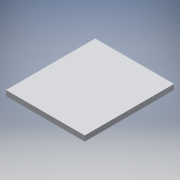
# Autodesk Inventor part: RSX Top
Saved by Autodesk Inventor 2016 (Build 200138000, 138)
## iProperties
Created: 2016-10-30
Part Number: RSX Top
Material: Aluminum 6061
Document SubType Name: Modeling
Designer: eschr_000
Density: 2.7 g/cm^3
Appearance: Aluminum - Flat
Author: eschr_000
Autodesk Inventor part; units mm, degrees
ref_plane "YZ Plane" through (0, 0, 0) normal (1, 0, 0) x (0, 1, 0)
ref_plane "XZ Plane" through (0, 0, 0) normal (0, 1, 0) x (-1, 0, 0)
ref_plane "XY Plane" through (0, 0, 0) normal (0, 0, 1) x (1, 0, 0)
sketch "Sketch1" plane through (0, 0, 0) normal (0, 1, 0) x (-1, 0, 0)
  line L0 (0, 0) -> (190.5, 0)
  line L1 (190.5, 0) -> (190.5, -215.9)
  line L2 (190.5, -215.9) -> (0, -215.9)
  line L3 (0, -215.9) -> (0, 0)
  dimension "d0" = 215.9
  dimension "d1" = 190.5
  constraints: 8 end point, 2 parallel, 1 horizontal, 1 perpendicular
  measures "d0" distance of L2.end L0.start
  measures "d1" distance of L0.start L0.end
extrude "Extrusion1" add sketch "Sketch1" along normal blind 12.7
sketch "Sketch2" plane through (0, 0, 0) normal (0, -1, 0) x (1, 0, 0)
  line L0 (-190.5, 0) -> (0, 0) construction
  line L1 (0, -215.9) -> (-190.5, -215.9) construction
  line L2 (0, 0) -> (-190.5, 0)
  line L3 (-190.5, 0) -> (-190.5, -215.9) construction
  line L4 (-190.5, -215.9) -> (0, -215.9)
  line L5 (0, -215.9) -> (0, 0) construction
  line L6 (-184.15, -209.55) -> (-184.15, -6.35)
  line L7 (-184.15, -6.35) -> (-6.35, -6.35)
  line L8 (-6.35, -6.35) -> (-6.35, -209.55)
  line L9 (-6.35, -209.55) -> (-184.15, -209.55)
  line L10 (-177.8, -203.2) -> (-12.7, -203.2)
  line L11 (-12.7, -12.7) -> (-63.5, -12.7)
  line L12 (-63.5, -12.7) -> (-63.5, -120.65)
  line L13 (-63.5, -120.65) -> (-12.7, -120.65)
  line L14 (-12.7, -120.65) -> (-12.7, -12.7)
  line L15 (-69.85, -120.65) -> (-69.85, -12.7)
  line L16 (-127, -6.35) -> (-6.35, -6.35)
  line L17 (-6.35, -6.35) -> (-6.35, -127)
  line L18 (-12.7, -127) -> (-127, -127)
  line L19 (-127, -127) -> (-177.8, -127)
  line L20 (-69.85, -120.65) -> (-177.8, -120.65)
  line L21 (-12.7, -12.7) -> (-63.5, -12.7)
  line L22 (-69.85, -12.7) -> (-177.8, -12.7)
  line L23 (-12.7, -203.2) -> (-12.7, -127)
  line L24 (-12.7, -120.65) -> (-12.7, -12.7)
  line L25 (-177.8, -12.7) -> (-177.8, -120.65)
  line L26 (-177.8, -127) -> (-177.8, -203.2)
  dimension "d4" = 6.35
  dimension "d8" = 6.35
  dimension "d11" = 107.95
  dimension "d12" = 107.95
  constraints: 50 end point, 14 parallel, 12 perpendicular, 2 horizontal, 4 other
  measures "d4" distance between parallel lines of L3 L6
  measures "d8" distance between parallel lines of L12 L15
  measures "d11" distance of L15.end L22.end
  measures "d12" distance of L22.end L20.end
extrude "Extrusion2" cut sketch "Sketch2" against normal blind 6.35
body "Solid1"
